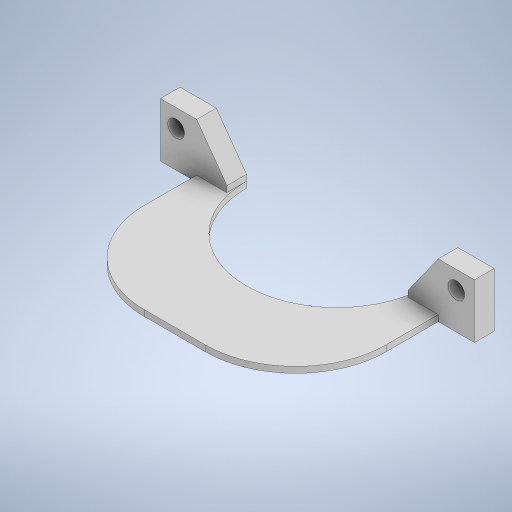
# Autodesk Inventor part: PartsForRaspibase
Saved by Autodesk Inventor 2024.2 (Build 282272000, 272)
## iProperties
Created: 2024-04-03
Part Number: PartsForRaspibase
Material: 一般
Document SubType Name: Modeling
Designer: yukin
Density: 1 g/cm^3
Appearance: 既定
Author: yukin
Autodesk Inventor part; units mm, degrees
ref_plane "YZ Plane" through (0, 0, 0) normal (1, 0, 0) x (0, 1, 0)
ref_plane "XZ Plane" through (0, 0, 0) normal (0, 1, 0) x (-1, 0, 0)
ref_plane "XY Plane" through (0, 0, 0) normal (0, 0, 1) x (1, 0, 0)
sketch "スケッチ1" plane through (0, 0, 0) normal (0, 1, 0) x (-1, 0, 0)
  line L0 (0, 0) -> (40, 0)
  line L1 (40, 0) -> (40, -26.8558)
  line L2 (40, -26.8558) -> (0, -26.8558)
  line L3 (0, -26.8558) -> (0, 0)
  circle A0 centre (20, -26.8558) radius 15
  line L4 (20, -26.8558) -> (20, 0)
  line L5 (40, -23.6058) -> (40, -26.8558)
  line L6 (0, -23.6058) -> (0, -26.8558)
  circle A1 centre (20, -26.8558) radius 17
  line L7 (40, -26.8558) -> (46, -26.8558)
  line L8 (46, -26.8558) -> (46, -23.6058)
  line L9 (46, -23.6058) -> (40, -23.6058)
  line L10 (40, -23.6058) -> (40, -26.8558)
  line L11 (0, -23.6058) -> (0, -26.8558)
  line L12 (0, -26.8558) -> (-6, -26.8558)
  line L13 (-6, -26.8558) -> (-6, -23.6058)
  line L14 (-6, -23.6058) -> (0, -23.6058)
  line L15 (0, -23.6058) -> (0, -26.8558)
  point P0 (35, -26.8558)
  point P1 (5, -26.8558)
  dimension "d0" = 40
  dimension "d1" = 30
  dimension "d16" = 34
  dimension "d18" = 6
  dimension "d19" = 3.25
  constraints: 32 end point, 5 symmetric about line, 4 parallel, 2 centre point, 2 horizontal, 2 midpoint, 2 perpendicular, 1 coincident
  measures "d0" distance of L1.end L2.end
  measures "d1" diameter of A0
  measures "d16" diameter of A1
  measures "d18" distance of L9.end L8.end
  measures "d19" distance of L8.end L7.end
extrude "押し出し1" add sketch "スケッチ1" along normal blind 1 contours L0 L4 A1 L2 L3 | L0 L1 L2 A1 L4 | A1 L2 A0 L4 | L4 A0 L2 A1 | L4 L2 A0 | A0 L2 L4
fillet "フィレット1" radius 15 2 edges at (-40, 0.5, 0) (0, 0.5, 0)
extrude "押し出し4" add sketch "スケッチ1" along normal blind 9 contours L3 L12 L13 L14 | L9 L8 L7 L1
sketch "スケッチ7" plane through (6, 0, -26.8558) normal (0, 0, -1) x (-1, 0, 0)
  circle A0 centre (3, 6) radius 1.375
  line L0 (6, 1) -> (6, 9) projected
  line L1 (0, 9) -> (6, 9) projected
  circle A1 centre (49.4019, 6) radius 1.375
  line L2 (46, 9) -> (52, 9) projected
  line L3 (52, 0) -> (52, 9) projected
  point P0 (6, 0)
  point P1 (3, 9)
  point P2 (52, 4.5)
  dimension "d22" = 2.75
  dimension "d23" = 3
  dimension "d24" = 3
  dimension "d25" = 2.75
  dimension "d26" = 3
  dimension "d27" = 3
  constraints: 2 centre point, 2 midpoint
  measures "d22" diameter of A0
  measures "d23" distance from line of L0 A0.centre
  measures "d24" distance of A0.centre point (3, 9)
  measures "d25" diameter of A1
  measures "d26" distance from line of A1.centre L2
  measures "d27" distance of point (52, 4.5) A1.centre
extrude "押し出し5" cut sketch "スケッチ7" against normal blind 6
extrude "押し出し6" cut sketch "スケッチ1" along normal blind 1 contours L4 L2 A0 | A0 L2 L4
sketch "スケッチ9" plane through (6, 9, -26.8558) normal (0, 0, -1) x (-1, 0, 0)
  line L0 (6, -8) -> (6, 0) projected
  line L1 (6, -8) -> (11, -8)
  line L2 (11, -8) -> (11, -7)
  line L3 (11, -7) -> (6, -7)
  line L4 (6, -7) -> (6, -8)
  line L5 (6, 0) -> (11, -7)
  line L6 (41, -8) -> (41, -9) projected
  line L7 (52, 0) -> (46, 0) projected
  line L8 (46, -8) -> (46, 0) projected
  line L9 (46, -8) -> (41, -8)
  line L10 (41, -8) -> (41, -7)
  line L11 (41, -7) -> (46, -7)
  line L12 (46, -7) -> (46, -8)
  line L13 (46, 0) -> (41, -7)
  point P0 (6, -9)
  dimension "d32" = 5
  dimension "d33" = 1
  dimension "d38" = 5
  constraints: 20 end point, 4 parallel, 2 horizontal, 2 perpendicular
  measures "d32" distance of L3.end L2.end
  measures "d33" distance of L2.end L1.end
  measures "d38" distance of L10.end L11.end
extrude "押し出し7" add sketch "スケッチ9" against normal blind 3.25
